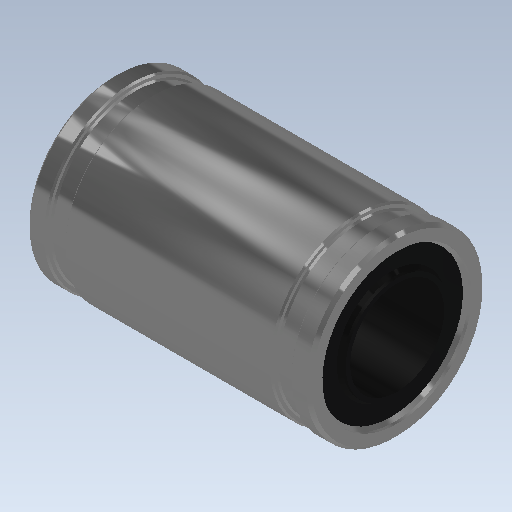
# Autodesk Inventor part: LM8UU 8mm Linear Bearing
Saved by Autodesk Inventor 2020.2 (Build 242310000, 310)
## iProperties
Created: 2012-04-01
Part Number: LM8UU 8mm Linear Bearing
Material: Ogólny
Document SubType Name: Modeling
Designer: Beau-James
Density: 1 g/cm^3
Appearance: Chrom - czarny polerowany
Author: Beau-James
Autodesk Inventor part; units mm, degrees
ref_plane "YZ Plane" through (0, 0, 0) normal (1, 0, 0) x (0, 1, 0)
ref_plane "XZ Plane" through (0, 0, 0) normal (0, 1, 0) x (-1, 0, 0)
ref_plane "XY Plane" through (0, 0, 0) normal (0, 0, 1) x (1, 0, 0)
sketch "Sketch1" plane through (0, 0, 0) normal (0, 0, 1) x (1, 0, 0)
  line L0 (0, 0) -> (23.5, 0)
  line L1 (0, 0) -> (0, 4) construction
  line L2 (0, 4) -> (23.5, 4) construction
  line L3 (0, 0) -> (0, 7.5) construction
  line L4 (0, 7.5) -> (23.5, 7.5) construction
  line L5 (23.5, 7.5) -> (23.5, 0) construction
  line L6 (0, 7.5) -> (23.5, 7.5)
  line L7 (1.5875, 7.5) -> (1.5875, 6.992)
  line L8 (1.5875, 6.992) -> (3.175, 6.992)
  line L9 (3.175, 6.992) -> (3.175, 7.5)
  line L10 (0, 7.5) -> (24, 7.5)
  line L11 (0, 4) -> (24, 4)
  line L12 (24, 4) -> (24, 4.3755)
  line L13 (24, 4.3755) -> (23.5, 4.3755)
  line L14 (23.5, 6.35) -> (24, 6.35)
  line L15 (24, 6.35) -> (24, 7.5)
  line L16 (0, 7.5) -> (0, 6.35)
  line L17 (0, 4) -> (0, 4.3755)
  line L18 (0.5103, 4.3755) -> (0, 4.3755)
  line L19 (0.5103, 4.3755) -> (0.5103, 6.35)
  line L20 (0.5103, 6.35) -> (0, 6.35)
  line L21 (24, 7.5) -> (22.3998, 7.5)
  line L22 (22.3998, 7.5) -> (22.3998, 6.992)
  line L23 (22.3998, 6.992) -> (20.7996, 6.992)
  line L24 (20.7996, 6.992) -> (20.7996, 7.5)
  line L25 (0, 7.5) -> (0, 6.35)
  line L26 (0, 6.35) -> (0.5103, 6.35)
  line L27 (0.5103, 6.35) -> (0.5103, 4.3755)
  line L28 (0, 4) -> (24, 4)
  line L29 (23.5, 6.35) -> (23.5, 4.3755)
  line L30 (22.3998, 7.5) -> (24, 7.5)
  line L31 (24, 7.5) -> (24, 6.35)
  line L32 (22.3998, 7.5) -> (22.3998, 6.992)
  line L33 (22.3998, 6.992) -> (20.7996, 6.992)
  line L34 (20.7996, 6.992) -> (20.7996, 7.5)
  dimension "d0" = 23.5
  dimension "d1" = 4
  dimension "d2" = 7.5
  dimension "d3" = 0.508
  dimension "d4" = 24
  dimension "d5" = 24
  dimension "d6" = 1.6002
  dimension "d7" = 1.6002
  constraints: 70 end point, 16 perpendicular, 11 point on line, 9 collinear, 3 parallel, 1 horizontal
  measures "d0" distance of L0.start L0.end
  measures "d1" distance of L0.start L1.end
  measures "d2" distance of L0.start L3.end
  measures "d3" distance of L7.start L7.end
  measures "d4" distance of L3.end L10.end
  measures "d5" distance of L1.end L11.end
  measures "d6" distance of L10.end L21.end
  measures "d7" distance of L22.end L23.end
revolve "Revolution1" add sketch "Sketch1" angle 360 about axis through (0, 0, 0) along (1, 0, 0) contours L6 L7 L8 L9 L24 L23 L22 L10 L15 L14 L29 L13 L12 L11 L17 L18 L19 L20 L16
chamfer "Chamfer1" distance 0.254 angle 45 6 edges at (24, -7.5, 0) (0, -7.5, 0) (23.5, -4.3755, 0) (23.5, -6.35, 0) (0.5103, -6.35, 0) (0.5103, -4.3755, 0)
chamfer "Chamfer2" distance 0.127 angle 45 8 edges at (3.175, -7.5, 0) (3.175, -6.992, 0) (22.3998, -7.5, 0) (22.3998, -6.992, 0) (1.5875, -6.992, 0) (20.7996, -6.992, 0) (20.7996, -7.5, 0) (1.5875, -7.5, 0)
body "Solid1"
